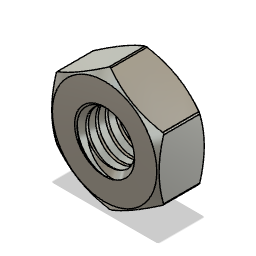
M3 Nut v2 (Autodesk Fusion 360 design; units mm, degrees)
Autodesk Fusion 360 part; units mm, degrees
sketch "Skizze1" plane through (0, 0, 0) normal (0, 0, 1) x (1, 0, 0)
  line L0 (-2.75, -1.5877) -> (0, -3.1754)
  line L1 (0, -3.1754) -> (2.75, -1.5877)
  line L2 (2.75, -1.5877) -> (2.75, 1.5877)
  line L3 (2.75, 1.5877) -> (0, 3.1754)
  line L4 (0, 3.1754) -> (-2.75, 1.5877)
  line L5 (-2.75, 1.5877) -> (-2.75, -1.5877)
  dimension "d3" = 2.75
  constraint vertical L5
  measures "d3" distance of origin L5
extrude "Extrusion1" add sketch "Skizze1" along normal mid plane 2.4
sketch "Skizze2" plane through (0, 0, 1.2) normal (0, 0, 1) x (1, 0, 0)
  line L0 (-2.75, 1.5877) -> (-2.75, -1.5877)
  line L1 (-2.75, -1.5877) -> (0, -3.1754)
  line L2 (0, -3.1754) -> (2.75, -1.5877)
  line L3 (2.75, -1.5877) -> (2.75, 1.5877)
  line L4 (2.75, 1.5877) -> (0, 3.1754)
  line L5 (0, 3.1754) -> (-2.75, 1.5877)
hole "Bohrung1" at (0, 0, 1.2) direction (0, 0, -1) diameter 2.529 end through all
thread "Gewinde1" "ISO Metric profile 3.0 M3x0.5 6H" major diameter 3.086 minor diameter 2.529 pitch 0.5 angle 60 modelled right hand crest width 0.1368 on face at (0.1259, -1.2582, -0.4) crest through (1.2645, 0, 1.075)
sketch "Skizze4" plane through (0, 0, 0) normal (1, 0, 0) x (0, 0, -1)
  line L0 (1.2, 1.5877) -> (1.2, 3.1754)
  line L1 (1.2, -3.1754) -> (1.2, -1.5877)
  line L2 (1.2, 3.1754) -> (-1.2, 3.1754)
  line L3 (0.9113, 3.1754) -> (1.2, 2.6754)
  line L4 (1.2, 3.1754) -> (0.9835, 3.0504) construction
  line L5 (1.2, 2.6754) -> (1.2, 0)
  line L6 (0.9113, 3.1754) -> (0, 3.1754)
  line L7 (0, 1.75) -> (0, 22.5) construction
  line L8 (-0.9113, 3.1754) -> (0, 3.1754)
  line L9 (-0.9113, 3.1754) -> (-1.2, 2.6754)
  line L10 (-1.2, 2.6754) -> (-1.2, 0)
  line L11 (-1.2, 0) -> (1.2, 0)
  line L12 (-1.2, 3.6754) -> (0, 3.6754)
  line L13 (1.2, 3.6754) -> (0, 3.6754)
  line L14 (1.2, 3.6754) -> (1.7, 2.8094)
  line L15 (1.7, 2.8094) -> (1.7, -0.5)
  line L16 (-1.7, -0.5) -> (1.7, -0.5)
  line L17 (-1.7, 2.8094) -> (-1.7, -0.5)
  line L18 (-1.2, 3.6754) -> (-1.7, 2.8094)
  line L19 (-1.2, 0) -> (-1.7, 0)
  line L20 (1.2, 0) -> (1.7, 0)
  line L21 (1.2, -1.5877) -> (1.2, 1.5877)
  line L22 (-1.75, 0) -> (-22.5, 0)
  dimension "d18" = 0.25
  dimension "d19" = 0.5
  dimension "d23" = 150
  constraint coincident L2 L3.start
  constraint coincident L0 L3.end
  constraint coincident L0.end L2.start
  constraint midpoint L2 L6.end
  constraint symmetric L3.start L7 L8.start
  constraint symmetric L3.end L7 L9.end
  constraint symmetric L5.end L7 L10.end
  constraint symmetric L6.end L7 L8.end
  constraint coincident L17 L19.end
  constraint perpendicular L17 L19
  constraint coincident L15 L20.end
  constraint perpendicular L15 L20
  constraint perpendicular L3 L4
  constraint coincident L3 L4.end
  constraint vertical L10
  constraint collinear L19 L22
  measures "d18" distance of L0.end L4.end
  measures "d23" angle of L3 L5
revolve "Drehen1" cut sketch "Skizze4" angle 360 about axis through (0, 0, 1.75) along (0, 0, 1) contours L0 L2 L5 L6 L8 L9 L10 L12 L13 L14 L15 L17 L18 L19 L20 L21 | L0 L2 L3
fillet "Abrundung1" radius 0.1 6 edges at (2.75, 1.5877, 0) (2.75, -1.5877, 0) (0, -3.1754, 0) (-2.75, -1.5877, 0) (0, 3.1754, 0) (-2.75, 1.5877, 0)
sketch "Skizze5" plane through (0, 0, 0) normal (1, 0, 0) x (0, 0, -1)
  line L0 (-1.2, 1.5328) -> (-0.9172, 1.25)
  line L1 (-0.9172, 1.25) -> (0, 1.25)
  line L2 (0, 1.75) -> (0, 22.5)
  line L3 (0, 1.25) -> (0, 0) construction
  line L4 (-0.9172, 1.25) -> (-1.2, 1.25) construction
  line L5 (-1.2, 1.25) -> (-1.0586, 1.3914) construction
  line L6 (-1.2, 1.5328) -> (-1.2, 0)
  line L7 (-1.2, 0) -> (0, 0)
  line L8 (0.9172, 1.25) -> (0, 1.25)
  line L9 (1.2, 1.5328) -> (0.9172, 1.25)
  line L10 (1.2, 1.5328) -> (1.2, 0)
  line L11 (1.2, 0) -> (0, 0)
  line L12 (-1.2, 2.6754) -> (-1.2, -2.6754)
  dimension "d28" = 1.25
  dimension "d29" = 0.2
  dimension "d31" = 45
  constraint horizontal L1
  constraint coincident L1.end L2
  constraint coincident L3.end L7.end
  constraint coincident L0 L5.end
  constraint perpendicular L0 L5
  constraint symmetric L0.start L2 L9.start
  constraint symmetric L0.end L2 L8.start
  constraint symmetric L1.end L2 L3.start
  constraint symmetric L2 L6.end L10.end
  constraint symmetric L2 L3.end L7.end
  constraint horizontal L7
  constraint vertical L6
  constraint horizontal L4
  constraint coincident L4.end L6
  constraint collinear L6 L12
  measures "d28" distance of L1.end L3.end
  measures "d29" distance of L4.end L5.end
  measures "d31" angle of L0 L6
revolve "Drehen2" cut sketch "Skizze5" angle 360 about axis through (0, 0, 1.75) along (0, 0, 1)
equation "HexWidth = 5.5 mm" comment "Side-to-side width"
equation "Height = 2.4 mm"
equation "d3 = HexWidth / 2"
equation "d4 = Height"
equation "ChamferDepth = 0.25 mm" comment "Corner chamfer depth"
equation "ChamferAngle = 30 deg" comment "Corner chamfer angle"
equation "ThreadChamferDepth = 0.2 mm"
equation "d18 = ChamferDepth"
equation "d19 = 2 * ChamferDepth"
equation "SideFillet = 0.1 mm" comment "Fillet of the sides"
equation "d22 = SideFillet"
equation "d23 = 180 deg - ChamferAngle"
equation "ThreadChamferAngle = 45 deg"
equation "CoreDrill = 2.5 mm" comment "Core drill size for the given thread. Used to compute the thread chamfer."
equation "d28 = CoreDrill / 2"
equation "d29 = ThreadChamferDepth"
equation "d31 = ThreadChamferAngle"
named bodies: "Nut"
